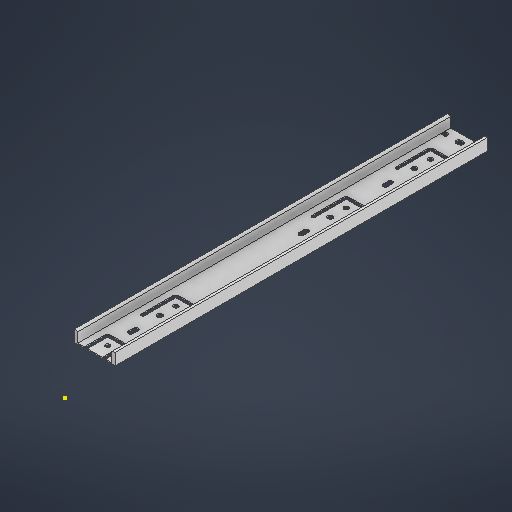
# Autodesk Inventor part: 1 часть направляшки 35
Saved by Autodesk Inventor 2025 (Build 290162000, 162)
## iProperties
Created: 2024-11-23
Part Number: 1 часть направляшки 35
Material: Типовые
Document SubType Name: Modeling
Designer: Phantom
Density: 1 g/cm^3
Appearance: По умолчанию
Author: Phantom
Autodesk Inventor part; units mm, degrees
ref_plane "YZ Plane" through (0, 0, 0) normal (1, 0, 0) x (0, 1, 0)
ref_plane "XZ Plane" through (0, 0, 0) normal (0, 1, 0) x (-1, 0, 0)
ref_plane "XY Plane" through (0, 0, 0) normal (0, 0, 1) x (1, 0, 0)
sketch "Эскиз1" plane through (0, 0, 0) normal (0, 0, 1) x (1, 0, 0)
  line L0 (0, 0) -> (-43, 0)
  line L1 (-43, 0) -> (-43, 11)
  line L2 (0, 0) -> (0, 11)
  line L3 (0, 11) -> (-3, 11)
  line L4 (-43, 11) -> (-40, 11)
  line L5 (-40, 11) -> (-40, 1)
  line L6 (-40, 1) -> (-3, 1)
  line L7 (-3, 1) -> (-3, 11)
  dimension "d0" = 43
  dimension "d1" = 11
  dimension "d2" = 11
  dimension "d3" = 3
  dimension "d4" = 10
  constraints: 16 end point, 5 perpendicular, 2 horizontal, 1 vertical
  measures "d0" distance of L0.start L0.end
  measures "d1" distance of L0.end L1.end
  measures "d2" distance of L0.start L2.end
  measures "d3" distance of L2.end L3.end
  measures "d4" distance of L4.end L5.end
extrude "Выдавливание1" add sketch "Эскиз1" along normal blind 400
sketch "Эскиз2" plane through (0, 0, 400) normal (0, 0, 1) x (1, 0, 0)
  line L0 (-40, 11) -> (-43, 11) projected
  line L1 (-43, 0) -> (0, 0) projected
  line L2 (-43, 11) -> (-34, 11)
  line L3 (-34, 11) -> (-34, 0)
  line L4 (-34, 0) -> (-43, 0)
  line L5 (-43, 0) -> (-43, 11)
  line L6 (0, 11) -> (-9, 11)
  line L7 (-9, 11) -> (-9, 0)
  line L8 (-9, 0) -> (0, 0)
  line L9 (0, 0) -> (0, 11)
  dimension "d7" = 9
  dimension "d8" = 9
  constraints: 16 end point, 4 parallel, 3 point on line, 2 horizontal, 2 perpendicular
  measures "d7" distance of L3.end L4.end
  measures "d8" distance of L8.end L7.end
extrude "Выдавливание2" add sketch "Эскиз2" against normal blind 88
sketch "Эскиз3" plane through (-43, 0, 0) normal (0, -1, 0) x (1, 0, 0)
  line L0 (0, 400) -> (43, 400) projected
  line L1 (0, 0) -> (0, 400) projected
  line L2 (0, 0) -> (43, 0) projected
  line L3 (43, 0) -> (43, 400) projected
  line L4 (21.5, 400) -> (21.5, -41)
  circle A0 centre (21.5, 289) radius 2.5
  circle A1 centre (21.5, 274) radius 2.25
  line L5 (21.5, 400) -> (28.5, 400)
  line L6 (21.5, 400) -> (14.5, 400)
  line L7 (14.5, 400) -> (14.5, -37.0777)
  line L8 (28.5, 400) -> (28.5, -41)
  line L9 (30, 298) -> (30, 254) construction
  line L10 (28.5, 296.5) -> (28.5, 267)
  line L11 (31.5, 266.5) -> (31.5, 296.5)
  arc A2 (31.5, 296.5) -> (28.5, 296.5) centre (30, 296.5) ccw
  line L12 (13, 298) -> (13, 252.5) construction
  line L13 (11.5, 296.5) -> (11.5, 266.5)
  line L14 (14.5, 267) -> (14.5, 296.5)
  arc A3 (14.5, 296.5) -> (11.5, 296.5) centre (13, 296.5) ccw
  line L15 (30, 254) -> (13, 254) construction
  line L16 (28.5, 267) -> (14.5, 267)
  line L17 (14.5, 264) -> (28.5, 264)
  arc A4 (28.5, 264) -> (31.5, 267) centre (28.75, 266.75) ccw
  arc A5 (11.5, 267) -> (14.5, 264) centre (14.25, 266.75) ccw
  circle A6 centre (21.5, 50) radius 2.5
  circle A7 centre (21.5, 35) radius 2.25
  line L18 (30, 59) -> (30, 15) construction
  line L19 (28.5, 57.5) -> (28.5, 28)
  line L20 (31.5, 27.5) -> (31.5, 57.5)
  arc A8 (31.5, 57.5) -> (28.5, 57.5) centre (30, 57.5) ccw
  line L21 (13, 59) -> (13, 13.5) construction
  line L22 (11.5, 57.5) -> (11.5, 27.5)
  line L23 (14.5, 28) -> (14.5, 57.5)
  arc A9 (14.5, 57.5) -> (11.5, 57.5) centre (13, 57.5) ccw
  line L24 (30, 15) -> (13, 15) construction
  line L25 (28.5, 28) -> (14.5, 28)
  line L26 (14.5, 25) -> (28.5, 25)
  arc A10 (28.5, 25) -> (31.5, 28) centre (28.75, 27.75) ccw
  arc A11 (11.5, 28) -> (14.5, 25) centre (14.25, 27.75) ccw
  circle A12 centre (21.5, 129) radius 2.5
  line L27 (14.5, 107) -> (14.5, 136.5)
  line L28 (28.5, 136.5) -> (28.5, 107)
  line L29 (11.5, 136.5) -> (11.5, 106.5)
  line L30 (31.5, 106.5) -> (31.5, 136.5)
  line L31 (13, 138) -> (13, 92.5) construction
  line L32 (30, 138) -> (30, 94) construction
  arc A13 (31.5, 136.5) -> (28.5, 136.5) centre (30, 136.5) ccw
  arc A14 (14.5, 136.5) -> (11.5, 136.5) centre (13, 136.5) ccw
  circle A15 centre (21.5, 114) radius 2.25
  arc A16 (28.5, 104) -> (31.5, 107) centre (28.75, 106.75) ccw
  line L33 (30, 94) -> (13, 94) construction
  line L34 (14.5, 104) -> (28.5, 104)
  arc A17 (11.5, 107) -> (14.5, 104) centre (14.25, 106.75) ccw
  line L35 (28.5, 107) -> (14.5, 107)
  line L36 (43, 7.5) -> (0, 7.5)
  line L37 (25, 7.5) -> (18, 7.5) construction
  line L38 (22.5, 10) -> (20.5, 10)
  line L39 (20.5, 5) -> (22.5, 5)
  arc A18 (22.5, 5) -> (22.5, 10) centre (22.5, 7.5) ccw
  arc A19 (20.5, 10) -> (20.5, 5) centre (20.5, 7.5) ccw
  line L40 (37.5326, 5.5358) -> (33.0331, 5.4647)
  line L41 (33.0331, 5.4647) -> (32.97, 9.4642)
  line L42 (32.97, 9.4642) -> (37.4694, 9.5353)
  line L43 (37.4694, 9.5353) -> (37.5326, 5.5358)
  line L44 (37.5326, 5.5358) -> (32.97, 9.4642) construction
  line L45 (33.0331, 5.4647) -> (37.4694, 9.5353) construction
  line L46 (5.4674, 5.5358) -> (9.9669, 5.4647)
  line L47 (9.9669, 5.4647) -> (10.03, 9.4642)
  line L48 (10.03, 9.4642) -> (5.5306, 9.5353)
  line L49 (5.5306, 9.5353) -> (5.4674, 5.5358)
  line L50 (5.4674, 5.5358) -> (10.03, 9.4642) construction
  line L51 (9.9669, 5.4647) -> (5.5306, 9.5353) construction
  circle A20 centre (21.5, 353) radius 2.5
  circle A21 centre (21.5, 338) radius 2.25
  line L52 (30, 362) -> (30, 318) construction
  line L53 (28.5, 360.5) -> (28.5, 331)
  line L54 (31.5, 330.5) -> (31.5, 360.5)
  arc A22 (31.5, 360.5) -> (28.5, 360.5) centre (30, 360.5) ccw
  line L55 (13, 362) -> (13, 316.5) construction
  line L56 (11.5, 360.5) -> (11.5, 330.5)
  line L57 (14.5, 331) -> (14.5, 360.5)
  arc A23 (14.5, 360.5) -> (11.5, 360.5) centre (13, 360.5) ccw
  line L58 (30, 318) -> (13, 318) construction
  line L59 (28.5, 331) -> (14.5, 331)
  line L60 (14.5, 328) -> (28.5, 328)
  arc A24 (28.5, 328) -> (31.5, 331) centre (28.75, 330.75) ccw
  arc A25 (11.5, 331) -> (14.5, 328) centre (14.25, 330.75) ccw
  line L61 (21.5, 70.4) -> (21.5, 79.6) construction
  line L62 (23.65, 72.55) -> (23.65, 77.45)
  line L63 (19.35, 77.45) -> (19.35, 72.55)
  arc A26 (19.35, 72.55) -> (23.65, 72.55) centre (21.5, 72.55) ccw
  arc A27 (23.65, 77.45) -> (19.35, 77.45) centre (21.5, 77.45) ccw
  line L64 (21.5, 149.4) -> (21.5, 158.6) construction
  line L65 (23.65, 151.55) -> (23.65, 156.45)
  line L66 (19.35, 156.45) -> (19.35, 151.55)
  arc A28 (19.35, 151.55) -> (23.65, 151.55) centre (21.5, 151.55) ccw
  arc A29 (23.65, 156.45) -> (19.35, 156.45) centre (21.5, 156.45) ccw
  line L67 (21.5, 309.4) -> (21.5, 318.6) construction
  line L68 (23.65, 311.55) -> (23.65, 316.45)
  line L69 (19.35, 316.45) -> (19.35, 311.55)
  arc A30 (19.35, 311.55) -> (23.65, 311.55) centre (21.5, 311.55) ccw
  arc A31 (23.65, 316.45) -> (19.35, 316.45) centre (21.5, 316.45) ccw
  line L70 (21.5, 373.4) -> (21.5, 382.6) construction
  line L71 (23.65, 375.55) -> (23.65, 380.45)
  line L72 (19.35, 380.45) -> (19.35, 375.55)
  arc A32 (19.35, 375.55) -> (23.65, 375.55) centre (21.5, 375.55) ccw
  arc A33 (23.65, 380.45) -> (19.35, 380.45) centre (21.5, 380.45) ccw
  point P0 (21.5, 271.75)
  point P1 (30, 275.25)
  point P2 (13, 275.25)
  point P3 (21.5, 254)
  point P4 (21.5, 52.5)
  point P5 (30, 36.25)
  point P6 (13, 36.25)
  point P7 (21.5, 15)
  point P8 (21.5, 69)
  point P9 (21.5, 131.5)
  point P10 (13, 115.25)
  point P11 (30, 115.25)
  point P12 (21.5, 111.75)
  point P13 (21.5, 94)
  point P14 (21.5, 128)
  point P15 (21.5, 128)
  point P16 (28.5, 296.5)
  point P17 (28.5, 267)
  point P18 (14.5, 267)
  point P19 (28.5, 107)
  point P20 (14.5, 107)
  point P21 (14.5, 136.5)
  point P22 (28.5, 28)
  point P23 (14.5, 28)
  point P24 (14.5, 57.5001)
  point P25 (28.5, 69)
  point P26 (21.5, 7.5)
  point P27 (21.5, 7.5)
  point P28 (35.2513, 7.5)
  point P29 (21.5, 335.75)
  point P30 (30, 339.25)
  point P31 (13, 339.25)
  point P32 (21.5, 318)
  point P33 (21.5, 75)
  point P34 (21.5, 159)
  point P35 (21.5, 154)
  point P36 (21.5, 304)
  point P37 (21.5, 314)
  point P38 (21.5, 366)
  point P39 (21.5, 378)
  point P40 (21.5, 331)
  point P41 (14.5, 296.5)
  point P42 (28.5, 264)
  point P43 (14.5, 264)
  point P44 (14.5, 264)
  point P45 (11.5, 267)
  point P46 (28.5, 264)
  point P47 (14.5, 107)
  point P48 (14.5, 25)
  point P49 (28.5, 28)
  point P50 (11.5, 28)
  point P51 (14.5, 25)
  point P52 (14.5, 331)
  point P53 (14.5, 360.5)
  point P54 (21.5, 5)
  dimension "d22" = 4.5
  dimension "d33" = 5
  dimension "d40" = 5
  dimension "d45" = 4.5
  dimension "d76" = 4.5
  dimension "d17" = 5
  dimension "d23" = 7
  dimension "d24" = 7
  dimension "d38" = 4.5
  dimension "d49" = 7.5
  dimension "d50" = 7
  dimension "d51" = 5
  dimension "d52" = 4.5
  dimension "d53" = 4
  dimension "d54" = 8
  dimension "d63" = 35
  dimension "d64" = 15
  dimension "d65" = 15
  dimension "d66" = 64
  dimension "d67" = 15
  dimension "d68" = 7
  dimension "d69" = 3
  dimension "d71" = 15
  dimension "d72" = 160
  dimension "d73" = 7
  dimension "d74" = 3
  dimension "d75" = 5
  dimension "d77" = 15
  dimension "d78" = 7
  dimension "d79" = 3
  dimension "d80" = 64
  dimension "d81" = 30
  dimension "d82" = 3
  dimension "d83" = 30
  dimension "d84" = 30
  dimension "d85" = 30
  dimension "d86" = 30
  dimension "d87" = 30
  dimension "d88" = 30
  dimension "d89" = 30
  dimension "d90" = 9.2
  dimension "d91" = 4.3
  dimension "d92" = 25
  dimension "d93" = 9.2
  dimension "d94" = 4.3
  dimension "d95" = 9.2
  dimension "d96" = 4.3
  dimension "d97" = 9.2
  dimension "d98" = 4.3
  dimension "d99" = 25
  dimension "d101" = 10
  dimension "d103" = 20
  dimension "d104" = 22
  dimension "d105" = 25
  dimension "d106" = 22
  dimension "d107" = 10
  dimension "d108" = 20
  dimension "d110" = 22
  dimension "d111" = 14
  dimension "d112" = 25
  dimension "d113" = 14
  dimension "d114" = 10
  dimension "d115" = 25
  dimension "d116" = 64
  dimension "d117" = 17
  dimension "d118" = 5
  dimension "d119" = 20.5
  constraints: 168 end point, 79 point on circle, 38 point on line, 36 tangent, 29 centre point, 20 parallel, 19 midpoint, 6 symmetric about line, 5 vertical alignment, 2 perpendicular, 1 horizontal, 17 other
  measures "d17" diameter of A0
  measures "d23" distance of L4.start L5.end
  measures "d24" distance of L4.start L6.end
  measures "d38" diameter of A7
  measures "d49" distance between parallel lines of L36 L2
  measures "d50" distance of L37.start L37.end
  measures "d51" diameter of A19
  measures "d52" distance of L40.start L40.end
  measures "d53" distance of L40.end L41.end
  measures "d54" distance from line of point (25, 7.5) L41
  measures "d63" distance from line of L2 A7.centre
  measures "d64" distance of A7.centre point (21.5, 50)
  measures "d65" distance between parallel lines of L38 L26
  measures "d66" distance of point (21.5, 114) point (21.5, 50)
  measures "d67" distance of point (21.5, 129) point (21.5, 114)
  measures "d68" distance from line of point (21.5, 114) L35
  measures "d69" distance between parallel lines of L34 L35
  measures "d71" distance of A0.centre point (21.5, 274)
  measures "d72" distance of point (21.5, 274) point (21.5, 114)
  measures "d73" distance from line of L16 point (21.5, 274)
  measures "d74" distance between parallel lines of L16 L17
  measures "d75" diameter of A20
  measures "d77" distance of A20.centre point (21.5, 338)
  measures "d78" distance from line of L59 point (21.5, 338)
  measures "d79" distance between parallel lines of L59 L60
  measures "d80" distance of point (21.5, 338) point (21.5, 274)
  measures "d81" distance of L22.start L22.end
  measures "d82" distance between parallel lines of L26 L25
  measures "d83" distance of L20.start L20.end
  measures "d84" distance of L29.start L29.end
  measures "d85" distance of L30.start L30.end
  measures "d86" distance of L11.start L11.end
  measures "d87" distance of L13.start L13.end
  measures "d88" distance of L56.start L56.end
  measures "d89" distance of L54.start L54.end
  measures "d90" distance of L61.start L61.end
  measures "d91" diameter of A27
  measures "d92" distance of point (21.5, 75) point (21.5, 50)
  measures "d93" distance of L64.start L64.end
  measures "d94" diameter of A29
  measures "d95" distance of L67.start L67.end
  measures "d96" diameter of A31
  measures "d97" distance of L70.start L70.end
  measures "d98" diameter of A33
  measures "d99" distance of point (21.5, 154) point (21.5, 129)
  measures "d101" distance from line of L11 A0.centre
  measures "d103" distance between parallel lines of L11 L13
  measures "d104" distance from line of L16 A0.centre
  measures "d105" distance of point (21.5, 314) A0.centre
  measures "d106" distance of point (21.5, 331) A20.centre
  measures "d107" distance from line of L54 A20.centre
  measures "d108" distance between parallel lines of L54 L56
  measures "d110" distance from line of L59 A20.centre
  measures "d112" distance of point (21.5, 378) A20.centre
  measures "d113" distance of L53.end L57.start
  measures "d114" distance from line of L60 point (21.5, 338)
  measures "d115" distance from line of L60 A20.centre
  measures "d116" distance of A0.centre A20.centre
  measures "d117" distance of A23.centre A22.centre
  measures "d118" distance from line of L2 point (21.5, 5)
  measures "d119" distance from line of L3 L39.end
extrude "Выдавливание3" cut sketch "Эскиз3" against normal blind 88 contours L7 A25 L56 A23 | L49 L48 L47 L36 | L36 L47 L46 L49 | A33 L71 A32 L4 | L4 A32 L72 A33 | L59 L4 L60 L7 | A22 L54 A24 L8 | L59 L8 L60 L4 | A20 L4 | L4 A20 | L7 A5 L13 A3 | A21 L4 | L4 A21 | L39 A19 L36 L4 | L4 L36 A18 L39 | A11 L22 A9 L7 | L7 L25 L4 L26 | A19 L38 L4 L36 | L43 L40 L41 L36 | L36 L41 L42 L43 | L16 L4 L17 L7 | A31 L68 A30 L4 | L4 A30 L69 A31 | L4 L38 A18 L36 | L4 L25 L8 L26 | A11 L22 | A2 L11 A4 L8 | L16 L8 L17 L4 | L13 A5 | L8 A8 L20 A10 | L7 A17 L29 A14 | A1 L4 | L4 A1 | A0 L4 | L4 A0 | L20 A10 | L7 L35 L4 L34 | A7 L4 | L4 A7 | A4 L11 | A29 L65 A28 L4 | L4 A28 L66 A29 | L4 L35 L8 L34 | A17 L29 | A13 L30 A16 L8 | A27 L62 A26 L4 | L4 A26 L63 A27 | A6 L4 | L4 A6 | A15 L4 | L4 A15 | A12 L4 | L4 A12 | L30 A16
fillet "Сопряжение3" radius 1 9 edges at (-14.5, 0.5, 267) (-9.9669, 0.5, 5.4647) (-5.4674, 0.5, 5.5358) (-5.5306, 0.5, 9.5353) (-10.03, 0.5, 9.4642) (-33.0331, 0.5, 5.4647) (-37.5326, 0.5, 5.5358) (-32.97, 0.5, 9.4642) (-37.4694, 0.5, 9.5353)
sketch "Эскиз4" plane through (0, 0, 400) normal (0, 0, 1) x (1, 0, 0)
  point P0 (0, 0)
sketch "Эскиз5" plane through (0, 0, 400) normal (0, 0, 1) x (1, 0, 0)
  line L0 (-40, 11) -> (-43, 11) projected
  line L1 (-43, 0) -> (0, 0) projected
  line L2 (-43, 11) -> (-40.5, 11)
  line L3 (-40.5, 11) -> (-40.5, 0)
  line L4 (-40.5, 0) -> (-43, 0)
  line L5 (-43, 0) -> (-43, 11)
  line L6 (0, 0) -> (0, 11) projected
  line L7 (0, 11) -> (-2.5, 11)
  line L8 (-2.5, 11) -> (-2.5, 0)
  line L9 (-2.5, 0) -> (0, 0)
  line L10 (0, 0) -> (0, 11)
  dimension "d55" = 2.5
  dimension "d56" = 2.5
  constraints: 16 end point, 4 parallel, 2 horizontal, 2 perpendicular, 2 point on line
  measures "d55" distance of L3.end L4.end
  measures "d56" distance of L9.end L8.end
extrude "Выдавливание4" cut sketch "Эскиз5" against normal through all
sketch "Эскиз6" plane through (0, 0, 0) normal (0, 0, -1) x (-1, 0, 0)
  line L0 (2.5, 11) -> (9, 11) projected
  line L1 (3, 11) -> (5.5, 11)
  line L2 (5.5, 11) -> (5.5, 0)
  line L3 (5.5, 0) -> (3, 0)
  line L4 (3, 0) -> (3, 11)
  line L5 (40, 11) -> (37.5, 11)
  line L6 (37.5, 11) -> (37.5, 0)
  line L7 (37.5, 0) -> (40, 0)
  line L8 (40, 0) -> (40, 11)
  point P0 (0, 0)
  dimension "d59" = 2.5
  dimension "d60" = 2.5
  constraints: 16 end point, 4 parallel, 3 point on line, 2 horizontal, 2 perpendicular
  measures "d59" distance of L2.end L3.end
  measures "d60" distance of L7.end L6.end
extrude "Выдавливание5" add sketch "Эскиз6" against normal through all
fillet "Сопряжение4" radius 6.5 2 edges at (-9, 11, 356) (-34, 11, 356)
sketch "Эскиз7" plane through (0, 0, 312) normal (0, 0, -1) x (-1, 0, 0)
  arc A0 (9, 4.5) -> (5.5, 10.2663) centre (2.5, 4.5) ccw projected
  line L0 (5.5, 10.2663) -> (5.5, 1) projected
  line L1 (9, 1) -> (5.5, 1) projected
  line L2 (9, 1) -> (9, 4.5) projected
  arc A1 (37.5, 10.2663) -> (34, 4.5) centre (40.5, 4.5) ccw projected
  line L3 (34, 4.5) -> (34, 1) projected
  line L4 (37.5, 1) -> (34, 1) projected
  line L5 (37.5, 1) -> (37.5, 10.2663) projected
  point P0 (0, 0)
extrude "Выдавливание6" cut sketch "Эскиз7" against normal through all
sketch "Эскиз8" plane through (-40.5, 0, 0) normal (0, -1, 0) x (1, 0, 0)
  arc A0 (12, 360.5) -> (9, 360.5) centre (10.5, 360.5) ccw projected
  line L0 (9, 360.5) -> (9, 407)
  line L1 (9, 407) -> (8, 407)
  line L2 (8, 407) -> (8, 400)
  line L3 (35, 400) -> (3, 400) projected
  line L4 (8, 400) -> (8, 391)
  line L5 (10, 389) -> (28.0494, 389)
  line L6 (30.0488, 390.95) -> (31, 429)
  line L7 (31, 429) -> (8, 407)
  arc A1 (8, 391) -> (10, 389) centre (10, 391) ccw
  arc A2 (28.0494, 389) -> (30.0488, 390.95) centre (28.0494, 391) ccw
  point P0 (40.5, 0)
  point P1 (8, 389)
  point P2 (30.275, 400)
  dimension "d123" = 11
  dimension "d124" = 2
  constraints: 14 end point, 5 tangent, 4 point on circle, 4 point on line, 2 centre point, 2 vertical, 1 equal radius, 1 horizontal, 1 perpendicular
  measures "d123" distance of L2.end point (8, 389)
  measures "d124" radius of A1
extrude "Выдавливание7" cut sketch "Эскиз8" against normal blind 10 contours A1 L4 L3 L0 | L0 L3 L6 A2 L5 A1
fillet "Сопряжение5" radius 2 2 edges at (-32.5, 0.5, 400) (-10.225, 0.5, 400)
sketch "Эскиз9" plane through (-37.5, 1, 0) normal (0, 1, 0) x (1, 0, 0)
  line L0 (7, -389) -> (25.0494, -389) projected
  line L1 (7, -389) -> (25, -389)
  line L2 (25, -389) -> (25, -388)
  line L3 (25, -388) -> (7, -388)
  line L4 (7, -388) -> (7, -389)
  point P0 (37.5, 0)
  constraints: 8 end point, 2 parallel, 1 horizontal, 1 perpendicular
extrude "Выдавливание8" add sketch "Эскиз9" along normal blind 7.5
fillet "Сопряжение6" radius 2 4 edges at (-30.5, 1, 388.5) (-30.5, 8.5, 388.5) (-12.5, 8.5, 388.5) (-12.5, 1, 388.5)
sketch "Эскиз10" plane through (0, 0, 400) normal (0, 0, 1) x (1, 0, 0)
  line L0 (-65, 32) -> (27, 32)
  line L1 (27, 32) -> (27, -9)
  line L2 (27, -9) -> (-65, -9)
  line L3 (-65, -9) -> (-65, 32)
  point P0 (0, 0)
  constraints: 8 end point, 2 parallel, 1 horizontal, 1 perpendicular
extrude "Выдавливание9" cut sketch "Эскиз10" against normal blind 50
